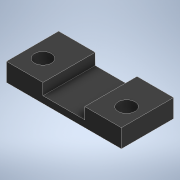
# Autodesk Inventor part: Stiftleiste_Halter
Saved by Autodesk Inventor 2021 (Build 250183000, 183)
## iProperties
Created: 2024-05-18
Part Number: Stiftleiste_Halter
Material: Generic
Document SubType Name: Modeling
Designer: Lukas
Density: 1 g/cm^3
Appearance: Default
Author: Lukas
Autodesk Inventor part; units mm, degrees
ref_plane "YZ Plane" through (0, 0, 0) normal (1, 0, 0) x (0, 1, 0)
ref_plane "XZ Plane" through (0, 0, 0) normal (0, 1, 0) x (-1, 0, 0)
ref_plane "XY Plane" through (0, 0, 0) normal (0, 0, 1) x (1, 0, 0)
sketch "Sketch1" plane through (0, 0, 0) normal (0, 0, 1) x (1, 0, 0)
  line L0 (-11, 1.75) -> (-4, 1.75)
  line L1 (-4, 1.75) -> (-4, -0.45)
  line L2 (-4, -0.45) -> (4, -0.45)
  line L3 (4, -0.45) -> (4, 1.75)
  line L4 (4, 1.75) -> (11, 1.75)
  line L5 (11, 1.75) -> (11, -1.75)
  line L6 (11, -1.75) -> (-11, -1.75)
  line L7 (-11, -1.75) -> (-11, 1.75)
  point P0 (0, 0)
  point P1 (0, -0.45)
  point P2 (-11, 0)
  point P3 (0, -1.75)
  dimension "d0" = 8
  dimension "d1" = 2.2
  dimension "d2" = 3.5
  dimension "d3" = 22
  constraints: 16 end point, 6 perpendicular, 3 midpoint, 2 point on line, 2 vertical alignment, 1 horizontal, 1 horizontal alignment
  measures "d0" distance of L1.end L2.end
  measures "d1" distance of L2.end L3.end
  measures "d2" distance of L4.end L5.end
  measures "d3" distance of L5.end L6.end
extrude "Extrusion1" add sketch "Sketch1" along normal blind 10
sketch "Sketch2" plane through (-11, -1.75, 0) normal (0, -1, 0) x (1, 0, 0)
  circle A0 centre (19, 6) radius 1.6
  circle A1 centre (3, 6) radius 1.6
  line L0 (0, 0) -> (22, 0) projected
  point P0 (11, 0)
  dimension "d6" = 6
  dimension "d7" = 16
  dimension "d8" = 8
  dimension "d9" = 3.2
  constraints: 2 centre point, 1 equal radius, 1 horizontal alignment
  measures "d6" distance from line of L0 A0.centre
  measures "d7" distance of A1.centre A0.centre
  measures "d8" horizontal distance of point (11, 0) A0.centre
  measures "d9" diameter of A0
extrude "Extrusion2" cut sketch "Sketch2" against normal through all
equation "\"d8\" = 0.5 * d7"
body "Solid1"
